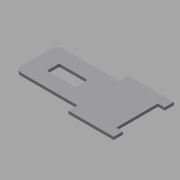
# Autodesk Inventor part: metal uc2
Saved by Autodesk Inventor 2017 (Build 210142000, 142)
## iProperties
Created: 2017-03-16
Part Number: metal uc2
Material: Generic
Document SubType Name: Modeling
Designer: Win10
Density: 1 g/cm^3
Appearance: Default
Author: Win10
Autodesk Inventor part; units mm, degrees
ref_plane "YZ Plane" through (0, 0, 0) normal (1, 0, 0) x (0, 1, 0)
ref_plane "XZ Plane" through (0, 0, 0) normal (0, 1, 0) x (-1, 0, 0)
ref_plane "XY Plane" through (0, 0, 0) normal (0, 0, 1) x (1, 0, 0)
sketch "Sketch1" plane through (0, 0, 0) normal (0, 0, 1) x (1, 0, 0)
  arc A0 (0.3092, 1.825) -> (0.4092, 1.925) centre (0.3092, 1.925) ccw projected
  line L0 (-4.7208, 1.825) -> (0.3092, 1.825) projected
  arc A1 (-4.7208, 1.825) -> (-5.1708, 1.375) centre (-4.7208, 1.375) ccw projected
  line L1 (-5.1708, -1.375) -> (-5.1708, 1.375) projected
  arc A2 (-5.1708, -1.375) -> (-4.7208, -1.825) centre (-4.7208, -1.375) ccw projected
  line L2 (0.3092, -1.825) -> (-4.7208, -1.825) projected
  arc A3 (0.4092, -1.925) -> (0.3092, -1.825) centre (0.3092, -1.925) ccw projected
  line L3 (0.4092, -2.65) -> (0.4092, -1.925) projected
  line L4 (4.3792, -2.65) -> (0.4092, -2.65) projected
  line L5 (4.3792, -1.925) -> (4.3792, -2.65) projected
  line L6 (3.8792, -1.925) -> (4.3792, -1.925) projected
  arc A4 (3.7792, -1.825) -> (3.8792, -1.925) centre (3.8792, -1.825) ccw projected
  line L7 (3.7792, 1.825) -> (3.7792, -1.825) projected
  arc A5 (3.8792, 1.925) -> (3.7792, 1.825) centre (3.8792, 1.825) ccw projected
  line L8 (4.3792, 1.925) -> (3.8792, 1.925) projected
  line L9 (4.3792, 2.65) -> (4.3792, 1.925) projected
  line L10 (0.4092, 2.65) -> (4.3792, 2.65) projected
  line L11 (0.4092, 1.925) -> (0.4092, 2.65) projected
  arc A6 (-1.2558, -0.55) -> (-1.1558, -0.45) centre (-1.2558, -0.45) ccw projected
  line L12 (-3.6058, -0.55) -> (-1.2558, -0.55) projected
  arc A7 (-3.7058, -0.45) -> (-3.6058, -0.55) centre (-3.6058, -0.45) ccw projected
  line L13 (-3.7058, 0.45) -> (-3.7058, -0.45) projected
  arc A8 (-3.6058, 0.55) -> (-3.7058, 0.45) centre (-3.6058, 0.45) ccw projected
  line L14 (-1.2558, 0.55) -> (-3.6058, 0.55) projected
  arc A9 (-1.1558, 0.45) -> (-1.2558, 0.55) centre (-1.2558, 0.45) ccw projected
  line L15 (-1.1558, -0.45) -> (-1.1558, 0.45) projected
  arc A10 (3.8303, -1.825) -> (3.8792, -1.874) centre (3.8792, -1.825) ccw
  line L16 (3.8792, -1.874) -> (4.4303, -1.874)
  line L17 (4.4303, -1.874) -> (4.4303, -2.701)
  line L18 (4.4303, -2.701) -> (0.3582, -2.701)
  line L19 (0.3582, -2.701) -> (0.3582, -1.925)
  arc A11 (0.3582, -1.925) -> (0.3092, -1.876) centre (0.3092, -1.925) ccw
  line L20 (0.3092, -1.876) -> (-4.7208, -1.876)
  arc A12 (-5.2218, -1.375) -> (-4.7208, -1.876) centre (-4.7208, -1.375) ccw
  line L21 (-5.2218, -1.375) -> (-5.2218, 1.375)
  arc A13 (-4.7208, 1.876) -> (-5.2218, 1.375) centre (-4.7208, 1.375) ccw
  line L22 (-4.7208, 1.876) -> (0.3092, 1.876)
  arc A14 (0.3092, 1.876) -> (0.3582, 1.925) centre (0.3092, 1.925) ccw
  line L23 (0.3582, 1.925) -> (0.3582, 2.701)
  line L24 (0.3582, 2.701) -> (4.4303, 2.701)
  line L25 (4.4303, 2.701) -> (4.4303, 1.874)
  line L26 (4.4303, 1.874) -> (3.8792, 1.874)
  arc A15 (3.8792, 1.874) -> (3.8303, 1.825) centre (3.8792, 1.825) ccw
  line L27 (3.8303, 1.825) -> (3.8303, -1.825)
  point P0 (0, 0)
  constraints: 24 end point, 12 point on circle, 6 centre point, 17 other
extrude "Extrusion1" add sketch "Sketch1" along normal blind 0.25 contours A0 L11 L10 L9 L8 A5 L7 A4 L6 L5 L4 L3 A3 L2 A2 L1 A1 L0 | A10 L16 L17 L18 L19 A11 L20 A12 L21 A13 L22 A14 L23 L24 L25 L26 A15 L27
sketch "Sketch2" plane through (0, 0, 0.25) normal (0, 0, 1) x (1, 0, 0)
  line L0 (3.8303, -1.825) -> (3.8303, 1.825) construction
  line L1 (3.8303, 1.5) -> (3.7053, 1.5)
  line L2 (3.7053, 1.5) -> (3.7053, -1.5)
  line L3 (3.7053, -1.5) -> (3.8303, -1.5)
  line L4 (3.8303, -1.5) -> (3.8303, 1.5)
  line L5 (3.8303, 1.5) -> (3.7053, -1.5) construction
  line L6 (3.7053, 1.5) -> (3.8303, -1.5) construction
  point P0 (0, 0)
  point P1 (3.7678, 0)
  dimension "d2" = 0.125
  dimension "d3" = 3
  constraints: 12 end point, 2 midpoint, 2 parallel, 1 collinear, 1 horizontal, 1 perpendicular
  measures "d2" distance of L3.end L2.end
  measures "d3" distance of L2.end L1.end
extrude "Extrusion2" add sketch "Sketch2" along normal blind 2
fillet "Fillet1" radius 0.05 68 edges at (3.8446, -1.8596, 0) (4.1548, -1.874, 0) (4.4303, -2.2875, 0) (2.3942, -2.701, 0) (0.3582, -2.313, 0) (0.3439, -1.8904, 0) (-2.2058, -1.876, 0) (-5.075, -1.7293, 0) (-5.2218, 0, 0) (-5.075, 1.7293, 0) (-2.2058, 1.876, 0) (0.3439, 1.8904, 0) (0.3582, 2.313, 0) (2.3942, 2.701, 0) (4.4303, 2.2875, 0) (4.1548, 1.874, 0) (3.8446, 1.8596, 0) (3.8303, 0, 0) (3.7678, -1.5, 0.25) (3.7053, 0, 0.25) (3.7678, 1.5, 0.25) (3.8303, 1.6625, 0.25) (3.8446, 1.8596, 0.25) (4.1548, 1.874, 0.25) (4.4303, 2.2875, 0.25) (2.3942, 2.701, 0.25) (0.3582, 2.313, 0.25) (0.3439, 1.8904, 0.25) (-2.2058, 1.876, 0.25) (-5.075, 1.7293, 0.25) (-5.2218, 0, 0.25) (-5.075, -1.7293, 0.25) (-2.2058, -1.876, 0.25) (0.3439, -1.8904, 0.25) (0.3582, -2.313, 0.25) (2.3942, -2.701, 0.25) (4.4303, -2.2875, 0.25) (4.1548, -1.874, 0.25) (3.8446, -1.8596, 0.25) (3.8303, -1.6625, 0.25) (3.7053, -1.5, 1.25) (3.7053, 0, 2.25) (3.7053, 1.5, 1.25) (3.8303, 1.5, 1.25) (3.8303, 0, 2.25) (3.8303, -1.5, 1.25) (4.4303, -2.701, 0.125) (0.3582, -2.701, 0.125) (4.4303, -1.874, 0.125) (4.4303, 2.701, 0.125) (4.4303, 1.874, 0.125) (0.3582, 2.701, 0.125) (-2.4308, -0.55, 0) (-2.4308, -0.55, 0.25) (-1.185, -0.5207, 0) (-1.1558, 0, 0) (-1.185, 0.5207, 0) (-2.4308, 0.55, 0) (-3.6765, 0.5207, 0) (-3.7058, 0, 0) (-3.6765, -0.5207, 0) (-3.6765, -0.5207, 0.25) (-3.7058, 0, 0.25) (-3.6765, 0.5207, 0.25) (-2.4308, 0.55, 0.25) (-1.185, 0.5207, 0.25) (-1.1558, 0, 0.25) (-1.185, -0.5207, 0.25)
body "Solid1"
